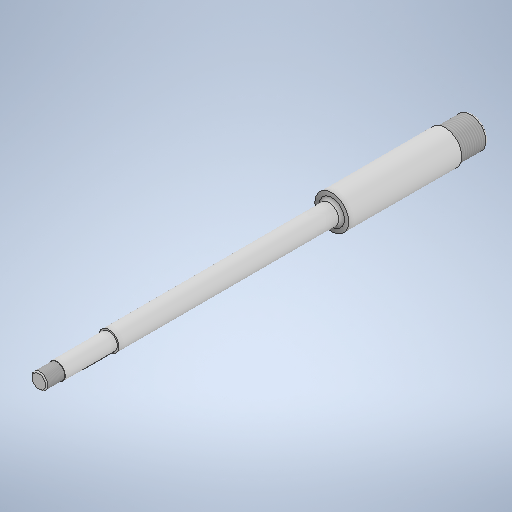
# Autodesk Inventor part: Lower Shaft
Saved by Autodesk Inventor 2025.2 (Build 292293000, 293)
## iProperties
Created: 2025-05-26
Part Number: Lower Shaft
Material: Generic
Document SubType Name: Modeling
Designer: abdal
Density: 1 g/cm^3
Appearance: Default
Author: abdal
Autodesk Inventor part; units mm, degrees
ref_plane "YZ Plane" through (0, 0, 0) normal (1, 0, 0) x (0, 1, 0)
ref_plane "XZ Plane" through (0, 0, 0) normal (0, 1, 0) x (-1, 0, 0)
ref_plane "XY Plane" through (0, 0, 0) normal (0, 0, 1) x (1, 0, 0)
sketch "Sketch1" plane through (0, 0, 0) normal (0, 0, 1) x (1, 0, 0)
  circle A0 centre (0, 0) radius 17.5
  dimension "d0" = 35
  constraints: 1 centre point, 1 coincident
  measures "d0" diameter of A0
extrude "Extrusion1" add sketch "Sketch1" along normal mid plane 725
sketch "Sketch3" plane through (0, 0, 362.5) normal (0, 0, 1) x (1, 0, 0)
  circle A0 centre (0, 0) radius 15
  circle A1 centre (0, 0) radius 17.5 projected
  dimension "d6" = 30
  constraints: 1 centre point, 1 coincident
  measures "d6" diameter of A0
extrude "Extrusion3" cut sketch "Sketch3" against normal blind 114
sketch "Sketch4" plane through (0, 0, 362.5) normal (0, 0, 1) x (1, 0, 0)
  circle A0 centre (0, 0) radius 14
  circle A1 centre (0, 0) radius 15 projected
  dimension "d9" = 28
  constraints: 1 centre point, 1 coincident
  measures "d9" diameter of A0
extrude "Extrusion4" cut sketch "Sketch4" against normal blind 22
thread "Thread1" size "M28x2" class "6g" standard "ANSI Metric M Profile" full length
sketch "Sketch5" plane through (0, 0, 362.5) normal (0, 0, 1) x (1, 0, 0)
  circle A0 centre (0, 0) radius 14 projected
extrude "Extrusion5" add sketch "Sketch5" along normal blind 10
fillet "Fillet1" radius 2 1 edges at (-14, 0, 372.5)
sketch "Sketch6" plane through (0, 0, 248.5) normal (0, 0, 1) x (1, 0, 0)
  line L0 (11.1074, -10.3393) -> (14.156, -14.3025) projected
  line L1 (7.1443, -13.3879) -> (11.1074, -10.3393) projected
  line L2 (7.1443, -13.3879) -> (10.1929, -17.351) projected
  line L3 (10.1929, -17.351) -> (14.156, -14.3025) projected
  point P0 (0, 0)
extrude "Extrusion6" cut sketch "Sketch6" along normal blind 55
sketch "Sketch7" plane through (0, 0, -362.5) normal (0, 0, -1) x (-1, 0, 0)
  circle A0 centre (0, 0) radius 17.5 projected
extrude "Extrusion7" cut sketch "Sketch7" against normal blind 17
sketch "Sketch8" plane through (0, 0, -345.5) normal (0, 0, -1) x (-1, 0, 0)
  circle A0 centre (0, 0) radius 30
  dimension "d21" = 60
  constraints: 1 centre point, 1 coincident
  measures "d21" diameter of A0
extrude "Extrusion8" add sketch "Sketch8" against normal blind 200
fillet "Fillet2" radius 5 1 edges at (-17.5, 0, -145.5)
sketch "Sketch9" plane through (0, 0, -345.5) normal (0, 0, -1) x (-1, 0, 0)
  circle A0 centre (0, 0) radius 17.5 projected
  circle A1 centre (0, 0) radius 27.5
  dimension "d25" = 55
  constraints: 1 centre point, 1 coincident
  measures "d25" diameter of A1
extrude "Extrusion9" add sketch "Sketch9" along normal blind 50 contours A0 | A1
sketch "Sketch10" plane through (0, 0, -345.5) normal (0, 0, -1) x (-1, 0, 0)
  line L0 (59.3657, -110.0033) -> (360.8409, -346.1125) projected
  arc A0 (360.8409, -346.1125) -> (422.4996, -267.3838) centre (0, 0) ccw projected
  line L1 (422.4996, -267.3838) -> (121.0244, -31.2746) projected
  arc A1 (121.0244, -31.2746) -> (65.5828, 106.4138) centre (0, 0) ccw projected
  line L2 (65.5828, 106.4138) -> (119.3218, 485.5536) projected
  arc A2 (119.3218, 485.5536) -> (20.3114, 499.5873) centre (0, 0) ccw projected
  line L3 (20.3114, 499.5873) -> (-33.4276, 120.4475) projected
  arc A3 (-33.4276, 120.4475) -> (-124.9485, 3.5894) centre (0, 0) ccw projected
  line L4 (-124.9485, 3.5894) -> (-480.1627, -139.4411) projected
  arc A4 (-480.1627, -139.4411) -> (-442.811, -232.2034) centre (0, 0) ccw projected
  line L5 (-442.811, -232.2034) -> (-87.5968, -89.1729) projected
  arc A5 (-87.5968, -89.1729) -> (59.3657, -110.0033) centre (0, 0) ccw projected
  line L6 (25.8741, -15.1833) -> (28.4468, -17.1982) projected
  line L7 (28.4468, -17.1982) -> (23.5141, -23.4965) projected
  line L8 (23.5141, -23.4965) -> (20.9414, -21.4816) projected
  arc A6 (25.8741, -15.1833) -> (20.9414, -21.4816) centre (0, 0) ccw projected
  line L9 (23.5141, -23.4965) -> (28.4468, -17.1982)
  line L10 (28.4468, -17.1982) -> (22.9358, -12.8821)
  line L11 (22.9358, -12.8821) -> (18.0031, -19.1804)
  line L12 (18.0031, -19.1804) -> (23.5141, -23.4965)
  point P0 (0, 0)
  dimension "d28" = 7
  dimension "d31" = 8
  constraints: 8 end point, 3 equal length, 1 perpendicular
  measures "d28" distance of L10.end L6.end
  measures "d31" distance of L6.end L7.end
extrude "Extrusion10" cut sketch "Sketch10" against normal blind 100 contours L6 L7 L8 L12 L11 L10
thread "Thread2" size "M55x4" class "6g" standard "ANSI Metric M Profile" full length
fillet "Fillet3" radius 5 1 edges at (27.5, 0, -395.5)
body "Solid1"
